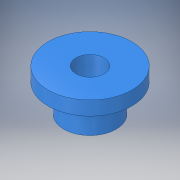
# Autodesk Inventor part: 3mmSpacer
Saved by Autodesk Inventor 2019.4 (Build 234330000, 330)
## iProperties
Created: 2021-02-02
Part Number: 3mmSpacer
Material: Generic
Document SubType Name: Modeling
Designer: Jorian Brusind
Density: 1 g/cm^3
Appearance: Cyan
Author: Jorian Brusind
Autodesk Inventor part; units mm, degrees
ref_plane "YZ Plane" through (0, 0, 0) normal (1, 0, 0) x (0, 1, 0)
ref_plane "XZ Plane" through (0, 0, 0) normal (0, 1, 0) x (-1, 0, 0)
ref_plane "XY Plane" through (0, 0, 0) normal (0, 0, 1) x (1, 0, 0)
sketch "Sketch1" plane through (0, 0, 0) normal (0, 1, 0) x (-1, 0, 0)
  circle A0 centre (0, 0) radius 3.75
  circle A1 centre (0, 0) radius 2
  dimension "d0" = 7.5
  dimension "d1" = 4
  constraints: 2 centre point, 2 coincident
  measures "d0" diameter of A0
  measures "d1" diameter of A1
extrude "Extrusion1" add sketch "Sketch1" along normal blind 4
sketch "Sketch2" plane through (0, 4, 0) normal (0, 1, 0) x (1, 0, 0)
  circle A0 centre (0, 0) radius 6
  circle A1 centre (0, 0) radius 2
  dimension "d4" = 12
  dimension "d5" = 4
  constraints: 2 centre point, 2 coincident
  measures "d4" diameter of A0
  measures "d5" diameter of A1
extrude "Extrusion2" add sketch "Sketch2" along normal blind 2
body "Solid1"
